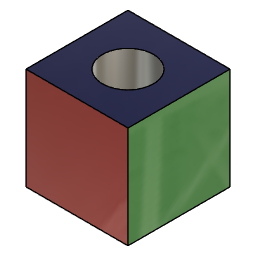
Workflow Template template v1 (Autodesk Fusion 360 archive; units mm, degrees)
design "WCS *"
Autodesk Fusion 360 part; units mm, degrees
sketch "WCS Profiles" plane through (0, 0, 0) normal (0, 0, 1) x (1, 0, 0)
  line L0 (20, 20) -> (-20, 20)
  line L1 (-20, 20) -> (-20, -20)
  line L2 (-20, -20) -> (20, -20)
  line L3 (20, -20) -> (20, 20)
  line L4 (20, 20) -> (-20, -20) construction
  line L5 (-20, 20) -> (20, -20) construction
  circle A0 centre (0, 0) radius 10
  dimension "d14" = 40
  dimension "d15" = 20
  constraint horizontal L0
  constraint perpendicular L0 L1
  constraint parallel L0 L2
  constraint parallel L1 L3
  constraint coincident L4 A0.centre
  constraint coincident L5 A0.centre
  constraint coincident A0.centre origin
  constraint equal L1 L2
  measures "d14" distance of L1.end L2.end
  measures "d15" diameter of A0
extrude "Extrude1" add sketch "WCS Profiles" along normal blind 40
